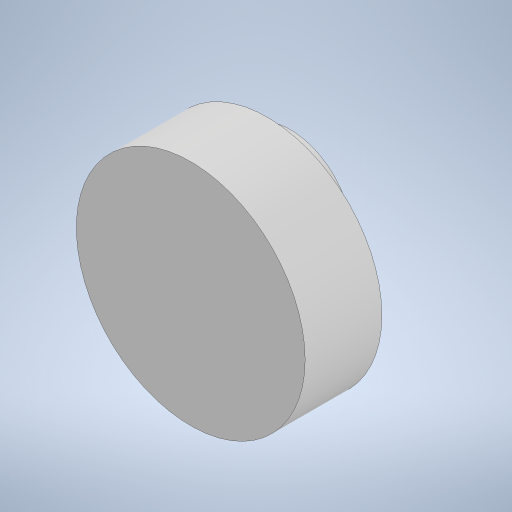
# Autodesk Inventor part: 감속기어1 - 상단 편심축
Saved by Autodesk Inventor 2023 (Build 270158000, 158)
## iProperties
Created: 2022-06-21
Part Number: 감속기어1 - 상단 편심축
Material: 일반
Document SubType Name: Modeling
Designer: user
Density: 1 g/cm^3
Appearance: 기본값
Author: user
Autodesk Inventor part; units mm, degrees
ref_plane "YZ Plane" through (0, 0, 0) normal (1, 0, 0) x (0, 1, 0)
ref_plane "XZ Plane" through (0, 0, 0) normal (0, 1, 0) x (-1, 0, 0)
ref_plane "XY Plane" through (0, 0, 0) normal (0, 0, 1) x (1, 0, 0)
sketch "스케치1" plane through (0, 0, 0) normal (0, 0, 1) x (1, 0, 0)
  circle A0 centre (2, 0) radius 7.45
  line L0 (0, 0) -> (2, 0)
  circle A1 centre (0, 0) radius 4
  line L1 (-2.6458, -3) -> (2.6458, -3)
  dimension "d1" = 14.9
  dimension "d2" = 2
  dimension "d3" = 8
  dimension "d4" = 3
  constraints: 4 end point, 2 centre point, 2 horizontal, 2 point on circle, 1 coincident
  measures "d1" diameter of A0
  measures "d2" distance of L0.start L0.end
  measures "d3" diameter of A1
  measures "d4" distance from line of L0.start L1
extrude "돌출1" add sketch "스케치1" along normal blind 5 contours A0 | A1 L1 | L1 A1
extrude "돌출2" add sketch "스케치1" against normal blind 3.5 contours A1 L1 picked at (1.0912, -0.393)
sketch "스케치3" plane through (2, 0, 0) normal (0, 0, -1) x (-1, 0, 0)
  arc A0 (4.6458, -3) -> (-0.6458, -3) centre (2, 0) ccw construction
  line L0 (-0.6458, -3) -> (4.6458, -3) construction
  circle A1 centre (2, 0) radius 5
  dimension "d12" = 10
  constraints: 1 centre point, 1 coincident
  measures "d12" diameter of A1
extrude "돌출3" add sketch "스케치3" along normal blind 1
